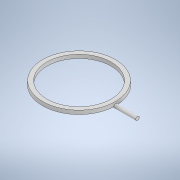
# Autodesk Inventor part: arm rings
Saved by Autodesk Inventor 2022 (Build 260153000, 153)
## iProperties
Created: 2022-03-14
Part Number: arm rings
Material: Generic
Document SubType Name: Modeling
Designer: mogje
Density: 1 g/cm^3
Appearance: Default
Author: mogje
Autodesk Inventor part; units mm, degrees
ref_plane "YZ Plane" through (0, 0, 0) normal (1, 0, 0) x (0, 1, 0)
ref_plane "XZ Plane" through (0, 0, 0) normal (0, 1, 0) x (-1, 0, 0)
ref_plane "XY Plane" through (0, 0, 0) normal (0, 0, 1) x (1, 0, 0)
sketch "Sketch1" plane through (0, 0, 0) normal (0, 1, 0) x (-1, 0, 0)
  arc A0 (-31.75, 0) -> (31.75, 0) centre (0, 0) ccw
  line L0 (0, 0) -> (-31.75, 0) construction
  line L1 (0, 0) -> (31.75, 0) construction
  line L2 (31.75, 0) -> (-31.75, 0)
  dimension "d0" = 31.75
  dimension "d1" = 180
  constraints: 6 end point, 2 point on circle, 1 centre point, 1 coincident
  measures "d0" radius of A0
  measures "d1" angle of L0 L1
revolve "Revolution1" add sketch "Sketch1" angle 180 about axis through (-31.75, 0, 0) along (1, 0, 0)
sketch "Sketch2" plane through (0, 0, 0) normal (0, -1, 0) x (1, 0, 0)
  line L0 (0, 0) -> (27.94, 0)
  circle A0 centre (0, 0) radius 27.94
  circle A1 centre (0, 0) radius 31.75
  dimension "d4" = 27.94
  constraints: 2 coincident, 2 end point, 1 centre point, 1 horizontal, 1 horizontal alignment, 2 other
  measures "d4" distance of L0.start L0.end
extrude "Extrusion1" cut sketch "Sketch2" against normal blind 3.175 keep common part
sketch "Sketch3" plane through (0, 0, 0) normal (1, 0, 0) x (0, 1, 0)
  circle A0 centre (0, 0) radius 1.5875
  dimension "d7" = 3.175
  constraints: 1 centre point, 1 coincident
  measures "d7" diameter of A0
extrude "Extrusion2" add sketch "Sketch3" along normal blind 50.8
sketch "Sketch4" plane through (0, 0, 0) normal (-1, 0, 0) x (0, 0, 1)
  circle A0 centre (0, 0) radius 1.5875 projected
  circle A1 centre (0, 0) radius 1.5875
  dimension "d10" = 3.175
  constraints: 1 centre point, 1 coincident
  measures "d10" diameter of A1
extrude "Extrusion3" cut sketch "Sketch4" against normal blind 28.575
sketch "Sketch5" plane through (0, 0, 0) normal (0, -1, 0) x (1, 0, 0)
  arc A0 (31.7103, 1.5875) -> (31.7103, -1.5875) centre (0, 0) ccw projected
  circle A1 centre (0, 0) radius 27.94 projected
  line L0 (27.0734, 12.56) -> (25.3453, 11.7583)
  line L1 (26.2309, -9.6221) -> (28.0193, -10.2782)
  arc A2 (26.2309, -9.6221) -> (25.3453, 11.7583) centre (0, 0) ccw
  arc A3 (28.0193, -10.2782) -> (27.0734, 12.56) centre (0, 0) ccw
  constraints: 6 point on circle, 4 end point, 2 centre point, 2 coincident, 1 other
sketch "Sketch6" plane through (0, 0, 0) normal (0, -1, 0) x (1, 0, 0)
  arc A0 (31.7103, 1.5875) -> (31.7103, -1.5875) centre (0, 0) ccw
  arc A1 (29.8078, -10.9342) -> (28.8015, 13.3617) centre (0, 0) ccw
  circle A2 centre (0, 0) radius 27.94
  line L0 (28.8015, 13.3617) -> (25.3453, 11.7583)
  line L1 (26.2309, -9.6221) -> (29.8078, -10.9342)
  arc A3 (26.2309, -9.6221) -> (25.3453, 11.7583) centre (0, 0) ccw
  point P0 (31.7103, -1.5875)
  point P1 (31.7103, 1.5875)
  constraints: 9 point on circle, 4 centre point, 4 end point, 2 coincident
extrude "Extrusion4" cut sketch "Sketch6" along normal blind 28.575 contours A1 A0 L1 A2 L0
extrude "Extrusion5" add sketch "Sketch5" against normal blind 1.5875 contours A1 L0 A3 L1
body "Solid1"
